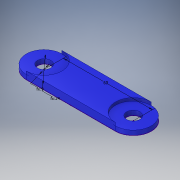
# Autodesk Inventor part: Middle_leg_a
Saved by Autodesk Inventor 2017 (Build 210142000, 142)
## iProperties
Created: 2016-06-08
Part Number: Middle_leg_a
Material: Generic
Document SubType Name: Modeling
Designer: alex-
Density: 1 g/cm^3
Appearance: Blue - Wall Paint - Glossy
Author: alex-
Autodesk Inventor part; units mm, degrees
ref_plane "YZ Plane" through (0, 0, 0) normal (1, 0, 0) x (0, 1, 0)
ref_plane "XZ Plane" through (0, 0, 0) normal (0, 1, 0) x (-1, 0, 0)
ref_plane "XY Plane" through (0, 0, 0) normal (0, 0, 1) x (1, 0, 0)
sketch "Sketch1" plane through (0, 0, 0) normal (0, 1, 0) x (-1, 0, 0)
  circle A0 centre (30, 0) radius 12
  circle A1 centre (-30, 0) radius 12
  line L0 (30, 12) -> (-30, 12)
  line L1 (30, -12) -> (-30, -12)
  circle A2 centre (30, 0) radius 4.5
  circle A3 centre (-30, 0) radius 4.5
  point P0 (0, 0)
  point P1 (0, 12)
  dimension "d5" = 60
  dimension "d6" = 24
  dimension "d7" = 9
  constraints: 4 centre point, 4 end point, 4 point on circle, 2 coincident, 2 equal radius, 2 horizontal alignment, 2 tangent, 1 horizontal, 1 midpoint, 1 parallel, 1 vertical alignment
  measures "d5" distance of A1.centre A0.centre
  measures "d6" diameter of A0
  measures "d7" diameter of A2
extrude "Extrusion2" add sketch "Sketch1" along normal blind 3 contours A0 | A1
extrude "Extrusion3" add sketch "Sketch1" along normal blind 5 contours A0 L1 A1 L0
equation "\"d6\" = sa_diameter"
equation "\"d7\" = s_shaft_dia"
equation "\"d8\" = b_mat_thickness - sa_thickness"
equation "\"d10\" = b_mat_thickness"
equation "\"sa_diameter\" = 24"
equation "\"s_shaft_dia\" = 9"
equation "\"b_mat_thickness\" = 5"
equation "\"sa_thickness\" = 2"
body "Solid2"
